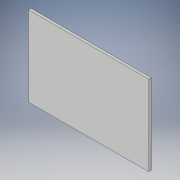
# Autodesk Inventor part: Teste
Saved by Autodesk Inventor 2018 (Build 220112000, 112)
## iProperties
Created: 2022-06-22
Part Number: Teste
Material: Generic
Document SubType Name: Modeling
Designer: Wesley Panazzolo
Density: 1 g/cm^3
Appearance: Default
Author: Wesley Panazzolo
Autodesk Inventor part; units mm, degrees
ref_plane "YZ Plane" through (0, 0, 0) normal (1, 0, 0) x (0, 1, 0)
ref_plane "XZ Plane" through (0, 0, 0) normal (0, 1, 0) x (-1, 0, 0)
ref_plane "XY Plane" through (0, 0, 0) normal (0, 0, 1) x (1, 0, 0)
sketch "Sketch1" plane through (0, 0, 0) normal (0, 0, 1) x (1, 0, 0)
  line L0 (-75, 50) -> (75, 50)
  line L1 (75, 50) -> (75, -50)
  line L2 (75, -50) -> (-75, -50)
  line L3 (-75, -50) -> (-75, 50)
  point P0 (0, 0)
  point P1 (0, 50)
  point P2 (75, 0)
  dimension "d0" = 150
  dimension "d1" = 100
  constraints: 8 end point, 2 midpoint, 2 parallel, 1 horizontal, 1 horizontal alignment, 1 perpendicular, 1 vertical alignment
  measures "d0" distance of L0.start L0.end
  measures "d1" distance of L0.end L1.end
extrude "Extrusion1" add sketch "Sketch1" along normal mid plane 3.17
body "Solid1"
